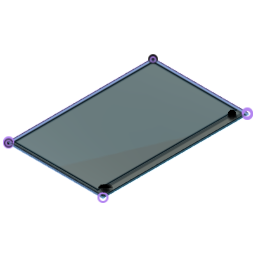
OpenBook Enclosure final (Autodesk Fusion 360 archive; units mm, degrees)
design "display"
Autodesk Fusion 360 part; units mm, degrees
sketch "Sketch1" plane through (0, 0, 0) normal (0, 0, 1) x (1, 0, 0)
  line L0 (-55.2571, 75.5392) -> (55.9429, 75.5392)
  line L1 (55.9429, 75.5392) -> (55.9429, -94.6608)
  line L2 (55.9429, -94.6608) -> (-55.2571, -94.6608)
  line L3 (-55.2571, -94.6608) -> (-55.2571, 75.5392)
  dimension "d1" = 111.2
  dimension "d2" = 170.2
  constraint horizontal L0
  constraint vertical L1
  constraint horizontal L2
  constraint vertical L3
  measures "d1" distance of L0.start L0.end
  measures "d2" distance of L0.start L2.end
extrude "Extrude1" add sketch "Sketch1" along normal blind 1.2 makes body 1
sketch "Sketch2" plane through (0, 0, 1.2) normal (0, 0, 1) x (-1, 0, 0)
  line L0 (55.2571, 94.6608) -> (-55.9429, 94.6608)
  line L1 (-55.9429, 94.6608) -> (-55.9429, -75.5392)
  line L2 (-55.9429, -75.5392) -> (55.2571, -75.5392)
  line L3 (55.2571, -75.5392) -> (55.2571, 94.6608)
sketch "Sketch3" plane through (0, 0, 1.2) normal (0, 0, 1) x (-1, 0, 0)
  line L0 (51.7571, -72.0392) -> (-46.1629, -72.0392)
  line L1 (-46.1629, -72.0392) -> (-46.1629, 91.1608)
  line L2 (-46.1629, 91.1608) -> (51.7571, 91.1608)
  line L3 (51.7571, 91.1608) -> (51.7571, -72.0392)
  line L4 (55.2571, -75.5392) -> (55.2571, 94.6608)
  line L5 (-55.9429, -75.5392) -> (55.2571, -75.5392)
  dimension "d8" = 97.92
  dimension "d9" = 163.2
  dimension "d10" = 3.5
  dimension "d11" = 3.5
  constraint horizontal L0
  constraint vertical L1
  constraint horizontal L2
  constraint vertical L3
  measures "d8" distance of L0.start L0.end
  measures "d9" distance of L0.start L2.end
  measures "d10" distance of L3 L4
  measures "d11" distance of L0 L5
sketch "Sketch5" plane through (0, 0, 0) normal (0, 0, 1) x (1, 0, 0)
  line L0 (-52.5571, 72.8392) -> (51.5329, 72.8392)
  line L1 (51.5329, -91.9608) -> (-52.5571, -91.9608)
  line L2 (-52.5571, -91.9608) -> (-52.5571, 72.8392)
  line L3 (-55.2571, 75.5392) -> (-55.2571, -94.6608)
  line L4 (55.9429, 75.5392) -> (-55.2571, 75.5392)
  line L5 (51.5329, 72.8392) -> (51.5329, 66.8392)
  line L6 (51.5329, -91.9608) -> (51.5329, -85.9608)
  line L7 (51.5329, -85.9608) -> (48.5329, -85.9608)
  line L8 (51.5329, 66.8392) -> (48.5329, 66.8392)
  line L9 (46.5329, 64.8392) -> (46.5329, -83.9608)
  arc A0 (46.5329, -83.9608) -> (48.5329, -85.9608) centre (48.5329, -83.9608) ccw
  arc A1 (48.5329, 66.8392) -> (46.5329, 64.8392) centre (48.5329, 64.8392) ccw
  line L10 (-55.2571, -94.6608) -> (55.9429, -94.6608)
  point P0 (46.5329, -85.9608)
  point P1 (46.5329, 66.8392)
  dimension "d14" = 164.8
  dimension "d15" = 104.09
  dimension "d16" = 2.7
  dimension "d17" = 2.7
  dimension "d19" = 6
  dimension "d21" = 6
  dimension "d22" = 5
  dimension "d23" = 5
  dimension "d24" = 2
  constraint horizontal L0
  constraint horizontal L1
  constraint vertical L2
  constraint perpendicular L0 L5
  constraint perpendicular L1 L6
  constraint perpendicular L6 L7
  constraint perpendicular L5 L8
  constraint perpendicular L7 L9
  constraint coincident P0 L7
  constraint coincident P0 L9
  constraint tangent L7 A0
  constraint tangent L9 A0
  constraint coincident P1 L8
  constraint coincident P1 L9
  constraint tangent L8 A1
  constraint tangent L9 A1
  constraint equal A0 A1
  measures "d14" distance of L0.start L1.end
  measures "d15" distance of L0.start L0.end
  measures "d16" distance of L2 L3
  measures "d17" distance of L0 L4
  measures "d19" distance of L0.end L5.end
  measures "d21" distance of L1.start L6.end
  measures "d22" distance of L6.end P0
  measures "d23" distance of L5.end P1
  measures "d24" radius of A0
sketch "Sketch12" plane through (0, 0, 0) normal (0, 0, 1) x (1, 0, 0)
  line L0 (-54.0571, 74.3392) -> (53.0329, 74.3392)
  line L1 (53.0329, -93.4608) -> (-54.0571, -93.4608)
  line L2 (-54.0571, -93.4608) -> (-54.0571, 74.3392)
  line L3 (-55.2571, -94.6608) -> (-55.2571, 75.5392)
  line L4 (-55.2571, 75.5392) -> (55.9429, 75.5392)
  line L5 (53.0329, 74.3392) -> (53.0329, 65.3392)
  line L6 (53.0329, 65.3392) -> (50.0329, 65.3392)
  line L7 (53.0329, -93.4608) -> (53.0329, -84.4608)
  line L8 (53.0329, -84.4608) -> (50.0329, -84.4608)
  line L9 (48.0329, -82.4608) -> (48.0329, 63.3392)
  arc A0 (50.0329, 65.3392) -> (48.0329, 63.3392) centre (50.0329, 63.3392) ccw
  arc A1 (48.0329, -82.4608) -> (50.0329, -84.4608) centre (50.0329, -82.4608) ccw
  point P0 (48.0329, 65.3392)
  point P1 (48.0329, -84.4608)
  dimension "d32" = 107.09
  dimension "d33" = 167.8
  dimension "d34" = 1.2
  dimension "d35" = 1.2
  dimension "d40" = 9
  dimension "d42" = 5
  dimension "d43" = 9
  dimension "d44" = 5
  dimension "d45" = 107.09
  dimension "d46" = 2
  dimension "d47" = 2
  constraint horizontal L0
  constraint horizontal L1
  constraint vertical L2
  constraint perpendicular L0 L5
  constraint perpendicular L5 L6
  constraint perpendicular L1 L7
  constraint perpendicular L7 L8
  constraint coincident P0 L6
  constraint coincident P0 L9
  constraint tangent L6 A0
  constraint tangent L9 A0
  constraint coincident P1 L8
  constraint coincident P1 L9
  constraint tangent L8 A1
  constraint tangent L9 A1
  measures "d32" distance of L0.start L0.end
  measures "d33" distance of L0.start L1.end
  measures "d34" distance of L2 L3
  measures "d35" distance of L0 L4
  measures "d40" distance of L0.end L5.end
  measures "d42" distance of L5.end P0
  measures "d43" distance of L1.start L7.end
  measures "d44" distance of L7.end P1
  measures "d45" distance of L1.start L1.end
  measures "d46" radius of A0
  measures "d47" radius of A1
copy_body "Body->Comp1" bodies 1 removing the originals makes body 2 in component "Component"
component "Component" placed x (1, 0, 0) y (0, 1, 0) z (0, 0, 1) at (0, 0, 0)
